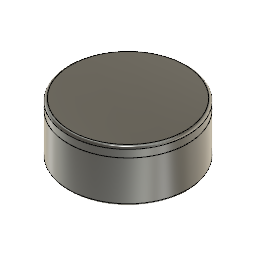
paperweight (Autodesk Fusion 360 design; units mm, degrees)
Autodesk Fusion 360 part; units mm, degrees
sketch "Sketch1" plane through (0, 0, 0) normal (0, 1, 0) x (1, 0, 0)
  line L0 (0, -45) -> (0, 23.1854)
  line L1 (0, 15) -> (-23, 15)
  line L2 (-24, 14) -> (-24, -2)
  line L3 (0, -2) -> (0, 15)
  arc A0 (-23, 15) -> (-24, 14) centre (-23, 14) ccw
  line L4 (-21, 9) -> (-8.5, 9)
  line L5 (-8.5, 9) -> (-8.5, 3)
  line L6 (-21, 0) -> (-21, 9)
  line L7 (-21, 0) -> (-21, -2)
  line L8 (-24, -2) -> (-21, -2)
  line L9 (-6, 3) -> (-8.5, 3)
  line L10 (0, -2) -> (-6, -2)
  line L11 (-6, -2) -> (-6, 3)
  line L12 (0, 3) -> (0, -2)
  dimension "d2" = 17
  dimension "d3" = 1
  dimension "d4" = 12.5
  dimension "d5" = 9
  constraint vertical L0
  constraint horizontal L1
  constraint vertical L2
  constraint horizontal L8
  constraint vertical L3
  constraint coincident L0 L1.start
  constraint tangent L2 A0
  constraint tangent L1 A0
  constraint horizontal L4
  constraint vertical L5
  constraint vertical L6
  constraint perpendicular L7 L8
  constraint perpendicular L5 L9
  constraint horizontal L10
  constraint vertical L11
  constraint vertical L12
  measures "d2" distance of L1.start L3.start
  measures "d3" radius of A0
  measures "d4" distance of L4.start L4.end
  measures "d5" distance of L4.start L6.start
revolve "Revolve1" add sketch "Sketch1" angle 360 about axis through (0, 0, 45) along (0, 0, -1) makes body 1
sketch "Sketch2" plane through (0, 0, -9) normal (0, 0, 1) x (-1, 0, 0)
  circle A0 centre (0, 0) radius 8.5
  circle A1 centre (0, 0) radius 21
  line L0 (19, 0) -> (5.8713, 18.0701)
  line L1 (5.8713, 18.0701) -> (-15.3713, 11.1679)
  line L2 (-15.3713, 11.1679) -> (-15.3713, -11.1679)
  line L3 (-15.3713, -11.1679) -> (5.8713, -18.0701)
  line L4 (5.8713, -18.0701) -> (19, 0)
  line L5 (14, 0) -> (4.3262, 13.3148)
  line L6 (4.3262, 13.3148) -> (-11.3262, 8.229)
  line L7 (-11.3262, 8.229) -> (-11.3262, -8.229)
  line L8 (-11.3262, -8.229) -> (4.3262, -13.3148)
  line L9 (4.3262, -13.3148) -> (14, 0)
  constraint coincident A0.centre A1.centre
extrude "Extrude1" cut sketch "Sketch2" against normal blind 4 contours L0 L1 L2 L3 L4 bodies 1
copy_body "Body->Comp1" bodies 1 removing the originals makes body 2 in component "Component"
sketch "Sketch1 (2)" plane through (0, 0, 0) normal (0, 1, 0) x (1, 0, 0) in component "Component'"
  line L0 (0, -11) -> (0, 18)
  line L1 (-24, -2) -> (-21, -2)
  line L2 (-21, -2) -> (-21, 0)
  line L3 (-21, 0) -> (-8.5, 0)
  line L4 (-8.5, 0) -> (-8.5, 3)
  line L5 (-6, 3) -> (-6, -2)
  line L6 (-6, -2) -> (0, -2)
  line L7 (-24, -2) -> (-24, -5)
  line L8 (-23, -6) -> (0, -6)
  line L9 (0, -2) -> (0, -6)
  line L10 (-6, 3) -> (-8.5, 3)
  arc A0 (-24, -5) -> (-23, -6) centre (-23, -5) ccw
  dimension "d9" = 12.5
  dimension "d10" = 1
  constraint vertical L0
  constraint horizontal L1
  constraint perpendicular L1 L2
  constraint perpendicular L2 L3
  constraint perpendicular L3 L4
  constraint perpendicular L3 L5
  constraint coincident L0 L6.end
  constraint perpendicular L0 L6
  constraint perpendicular L1 L7
  constraint coincident L0 L8.end
  constraint perpendicular L0 L8
  constraint perpendicular L4 L10
  constraint tangent L7 A0
  constraint tangent L8 A0
  measures "d9" distance of L2.end L3.end
  measures "d10" radius of A0
revolve "Revolve1'" add sketch "Sketch1 (2)" angle 360 about axis through (0, 0, 11) along (0, 0, -1) separate body makes body 3 in component "Component'"
sketch "Sketch2 (2)" plane through (0, 0, 0) normal (0, 0, -1) x (1, 0, 0) in component "Component'"
  circle A0 centre (0, 0) radius 21
  circle A1 centre (0, 0) radius 8.5
  line L0 (-19, 0) -> (-5.8713, -18.0701)
  line L1 (-5.8713, -18.0701) -> (15.3713, -11.1679)
  line L2 (15.3713, -11.1679) -> (15.3713, 11.1679)
  line L3 (15.3713, 11.1679) -> (-5.8713, 18.0701)
  line L4 (-5.8713, 18.0701) -> (-19, 0)
  line L5 (-14, 0) -> (-4.3262, -13.3148)
  line L6 (-4.3262, -13.3148) -> (11.3262, -8.229)
  line L7 (11.3262, -8.229) -> (11.3262, 8.229)
  line L8 (11.3262, 8.229) -> (-4.3262, 13.3148)
  line L9 (-4.3262, 13.3148) -> (-14, 0)
  constraint coincident A0.centre A1.centre
extrude "Extrude1'" cut sketch "Sketch2 (2)" against normal blind 4 contours L0 L1 L2 L3 L4 bodies 3 in component "Component'"
component "Component" placed x (1, 0, 0) y (0, 1, 0) z (0, 0, 1) at (0, 0, 0)
component "Component'" placed x (1, 0, 0) y (0, 1, 0) z (0, 0, 1) at (0, 0, 0) in component "Component"
